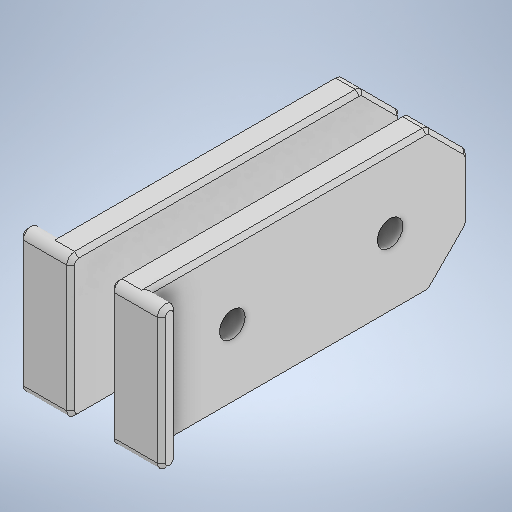
# Autodesk Inventor part: Fuß
Saved by Autodesk Inventor 2025.1 (Build 291241000, 241)
## iProperties
Created: 2024-11-26
Part Number: Fuß
Material: Generisch
Document SubType Name: Modeling
Designer: Kai Altwicker
Density: 1 g/cm^3
Appearance: Vorgabe
Author: Kai Altwicker
Autodesk Inventor part; units mm, degrees
ref_plane "YZ Plane" through (0, 0, 0) normal (1, 0, 0) x (0, 1, 0)
ref_plane "XZ Plane" through (0, 0, 0) normal (0, 1, 0) x (-1, 0, 0)
ref_plane "XY Plane" through (0, 0, 0) normal (0, 0, 1) x (1, 0, 0)
sketch "Skizze1" plane through (0, 0, 0) normal (0, 1, 0) x (-1, 0, 0)
  line L0 (9, 2) -> (-9, 2)
  line L1 (-9, 2) -> (-9, 0)
  line L2 (-9, 0) -> (-6, 0)
  line L3 (-6, 0) -> (-6, -40)
  line L4 (-6, -40) -> (-2.5, -40)
  line L5 (-2.5, -40) -> (-2.5, 0)
  line L6 (-2.5, 0) -> (2.5, 0)
  line L7 (2.5, 0) -> (2.5, -40)
  line L8 (2.5, -40) -> (6, -40)
  line L9 (6, -40) -> (6, 0)
  line L10 (6, 0) -> (9, 0)
  line L11 (9, 0) -> (9, 2)
  point P0 (0, 0)
  point P1 (0, 0)
  dimension "d0" = 3
  dimension "d1" = 5
  dimension "d2" = 2
  dimension "d3" = 3.5
  dimension "d4" = 40
  constraints: 24 end point, 6 equal length, 4 perpendicular, 3 parallel, 3 point on line, 1 coincident, 1 horizontal, 1 midpoint
  measures "d0" distance of L9.end L10.end
  measures "d1" distance of L5.end L6.end
  measures "d2" distance of L0.end L1.end
  measures "d3" distance of L3.end L4.end
  measures "d4" distance of L8.end L9.end
extrude "Extrusion1" add sketch "Skizze1" along normal blind 18
chamfer "Fasen3" distance 5 angle 45 4 edges at (-4.25, 18, -40) (4.25, 18, -40) (4.25, 0, -40) (-4.25, 0, -40)
fillet "Rundung3" radius 1 16 edges at (-4.25, 18, -35) (-4.25, 13, -40) (-4.25, 5, -40) (-4.25, 0, -35) (4.25, 0, -35) (4.25, 5, -40) (4.25, 13, -40) (4.25, 18, -35) (0, 18, 0) (7.5, 18, 0) (0, 18, 2) (-7.5, 18, 0) (-7.5, 0, 0) (0, 0, 2) (0, 0, 0) (7.5, 0, 0)
sketch "Skizze3" plane through (-6, 0, -34.5858) normal (-1, 0, 0) x (0, 0, 1)
  line L0 (34.5858, 1) -> (34.5858, 17) projected
  point P0 (34.5858, 0)
  point P1 (24.5858, 9)
  point P2 (4.5858, 9)
  point P3 (34.5858, 9)
  dimension "d28" = 10
  dimension "d29" = 20
  constraints: 2 horizontal alignment, 1 midpoint
  measures "d28" distance from line of L0 point (24.586, 9)
  measures "d29" distance of point (4.586, 9) point (24.586, 9)
hole "Bohrung2" at (-6, 9, -10) at (-6, 9, -30) direction (1, 0, 0) diameter 3.242 end through all thread size "M4x0.7" class "6H" standard "ISO Metric profile"
hole "Bohrung3" at (-6, 9, -10) at (-6, 9, -30) direction (1, 0, 0) diameter 4.5 depth 3.5 countersink diameter 9.4 countersink angle 90 clearance for "Flachkopfsenkschraube DIN EN ISO 2009" size "M4" standard "DIN"
sketch "Skizze4" plane through (-2.5, 1, 0) normal (1, 0, 0) x (0, 0, -1)
  line L0 (46.0679, 28.7323) -> (-6.5362, 28.7323)
  line L1 (-6.5362, 28.7323) -> (-6.5362, -10.7207)
  line L2 (-6.5362, -10.7207) -> (46.0679, -10.7207)
  line L3 (46.0679, -10.7207) -> (46.0679, 28.7323)
  point P0 (0, -1)
  constraints: 8 end point, 2 parallel, 1 horizontal, 1 perpendicular
extrude "Extrusion2" cut sketch "Skizze4" along normal up to surface (5 mm away)
chamfer "Fasen4" distance 0.5 angle 45 41 edges at (-2.5, 9, -40) (-2.5, 12.9685, -39.9239) (-2.5, 15.5, -37.5) (-2.5, 17.9239, -34.9685) (-2.5, 18, -16.7927) (-2.5, 0, -16.7927) (-2.5, 0.0761, -34.9685) (-2.5, 2.5, -37.5) (-2.5, 5.0315, -39.9239) (2.5, 5.0315, -39.9239) (2.5, 9, -40) (2.5, 12.9685, -39.9239) (2.5, 15.5, -37.5) (2.5, 17.9239, -34.9685) (2.5, 18, -16.7927) (2.5, 0, -16.7927) (2.5, 0.0761, -34.9685) (2.5, 2.5, -37.5) (6, 5.0315, -39.9239) (6, 2.5, -37.5) (6, 0.0761, -34.9685) (6, 0, -16.7932) (6, 9, -40) (6, 12.9685, -39.9239) (6, 15.5, -37.5) (6, 17.9239, -34.9685) (6, 18, -16.7932) (-6, 2.5, -37.5) (-6, 5.0315, -39.9239) (-6, 9, -40) (-6, 12.9685, -39.9239) (-6, 15.5, -37.5) (-6, 17.9239, -34.9685) (-6, 18, -16.7932) (-6, 0.0761, -34.9685) (-6, 0, -16.7932) (9, 9, 2) (9, 9, 0) (-9, 0.2927, 0.2927) (-9, 9, 0) (-9, 9, 2)
equation "\"d_tol\" = 0.3"
equation "\"d_wand\" = 1.5"
equation "\"b_rasp_pi\" = 56"
equation "\"w_kamera_hori\" = 66deg"
equation "\"l_rasp_pi\" = 85"
equation "\"w_kamera_vert\" = 41deg"
equation "\"r_rasp_pi\" = 3"
equation "\"D_oct\" = 3621.32034"
equation "\"D_hexadeca\" = 7541.00924"
equation "\"d_traeger\" = 625"
